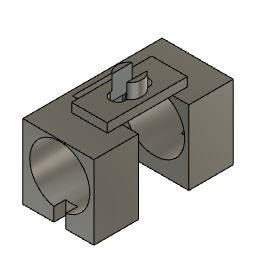
ENG_CRNK_mount-v2 v2-.25mm (Autodesk Fusion 360 design; units mm, degrees)
Autodesk Fusion 360 part; units mm, degrees
sketch "Sketch1" plane through (0, 0, 0) normal (0, 0, 1) x (1, 0, 0)
  line L0 (-39.3784, 42.4452) -> (-27.3784, 42.4452)
  line L1 (-27.3784, 42.4452) -> (-27.3784, 15.4452)
  line L2 (-27.3784, 15.4452) -> (-39.3784, 15.4452)
  line L3 (-39.3784, 15.4452) -> (-39.3784, 42.4452)
  dimension "d1" = 12
  dimension "d2" = 27
  constraint horizontal L0
  constraint vertical L1
  constraint horizontal L2
  constraint vertical L3
  measures "d1" distance of L0.start L0.end
  measures "d2" distance of L0.start L2.end
extrude "Extrude1" add sketch "Sketch1" along normal blind 3
sketch "Sketch2" plane through (0, 0, 3) normal (0, 0, 1) x (-1, 0, 0)
  line L0 (39.3784, -15.4452) -> (27.3784, -15.4452)
  line L1 (27.3784, -15.4452) -> (27.3784, -42.4452)
  line L2 (27.3784, -42.4452) -> (39.3784, -42.4452)
  line L3 (39.3784, -42.4452) -> (39.3784, -15.4452)
  circle A0 centre (33.3784, -28.9452) radius 4.25
  dimension "d5" = 8.5
  measures "d5" diameter of A0
extrude "Extrude2" add sketch "Sketch2" along normal blind 4.5 contours A0
sketch "Sketch3" plane through (0, 0, 0) normal (0, 0, -1) x (1, 0, 0)
  line L0 (-27.3784, -15.4452) -> (-39.3784, -15.4452)
  line L1 (-39.3784, -15.4452) -> (-39.3784, -42.4452)
  line L2 (-39.3784, -42.4452) -> (-27.3784, -42.4452)
  line L3 (-27.3784, -42.4452) -> (-27.3784, -15.4452)
  line L4 (-33.3784, -15.4452) -> (-30.8784, -15.4452) construction
  line L5 (-30.8784, -15.4452) -> (-35.8784, -15.4452)
  line L6 (-35.8784, -15.4452) -> (-35.8784, -42.4452)
  line L7 (-35.8784, -42.4452) -> (-30.8784, -42.4452)
  line L8 (-30.8784, -42.4452) -> (-30.8784, -15.4452)
  line L9 (-30.8784, -28.9452) -> (-30.8784, -24.9452) construction
  line L10 (-30.8784, -24.9452) -> (-35.8784, -24.9452)
  line L11 (-35.8784, -24.9452) -> (-35.8784, -32.9452)
  line L12 (-35.8784, -32.9452) -> (-30.8784, -32.9452)
  line L13 (-30.8784, -32.9452) -> (-30.8784, -24.9452)
  circle A0 centre (-33.3784, -32.9452) radius 2.5
  circle A1 centre (-33.3784, -24.9452) radius 2.5
  dimension "d8" = 2.5
  dimension "d9" = 5
  dimension "d10" = 4
  dimension "d11" = 8
  constraint midpoint L0 L4.start
  constraint perpendicular L3 L4
  constraint horizontal L5
  constraint vertical L6
  constraint horizontal L7
  constraint vertical L8
  constraint coincident L2 L6.end
  constraint midpoint L8 L9.start
  constraint coincident L8 L9.end
  constraint horizontal L10
  constraint vertical L11
  constraint horizontal L12
  constraint vertical L13
  constraint midpoint L12 A0.centre
  constraint coincident L12.end A0
  constraint midpoint L10 A1.centre
  constraint coincident L9.end A1
  measures "d8" distance of L4.start L4.end
  measures "d9" distance of L4.end L5.end
  measures "d10" distance of L9.start L9.end
  measures "d11" distance of L9.end L12.end
extrude "Extrude3" cut sketch "Sketch3" against normal blind 15 contours L10 A1 | L10 A1 | L6 L8 L11 L13 A0 A1 | L12 A0 | L12 A0
sketch "Sketch4" plane through (-35.8784, 0, 0) normal (1, 0, 0) x (0, 1, 0)
  line L0 (25.5083, 3) -> (24.9452, 3)
  line L1 (24.9452, 3) -> (24.9452, 0)
  line L2 (24.9452, 0) -> (32.9452, 0)
  line L3 (32.9452, 0) -> (32.9452, 3)
  line L4 (32.9452, 3) -> (32.3821, 3)
  line L5 (32.3821, 3) -> (32.3821, 7.5)
  line L6 (32.3821, 7.5) -> (25.5083, 7.5)
  line L7 (25.5083, 7.5) -> (25.5083, 3)
sketch "Sketch5" plane through (0, 0, 0) normal (0, 0, -1) x (1, 0, 0)
  line L0 (-35.8784, -32.9452) -> (-35.8784, -24.9452)
  arc A0 (-30.8784, -24.9452) -> (-35.8784, -24.9452) centre (-33.3784, -24.9452) ccw
  line L1 (-30.8784, -24.9452) -> (-30.8784, -32.9452)
  arc A1 (-35.8784, -32.9452) -> (-30.8784, -32.9452) centre (-33.3784, -32.9452) ccw
  line L2 (-27.3784, -15.4452) -> (-39.3784, -15.4452)
  line L3 (-39.3784, -15.4452) -> (-39.3784, -42.4452)
  line L4 (-39.3784, -42.4452) -> (-27.3784, -42.4452)
  line L5 (-27.3784, -42.4452) -> (-27.3784, -15.4452)
  line L6 (-39.3784, -42.4452) -> (-27.3784, -42.4452)
  line L7 (-27.3784, -42.4452) -> (-27.3784, -38.4452)
  line L8 (-27.3784, -38.4452) -> (-39.3784, -38.4452)
  line L9 (-39.3784, -38.4452) -> (-39.3784, -42.4452)
  line L10 (-39.3784, -15.4452) -> (-27.3784, -15.4452)
  line L11 (-27.3784, -15.4452) -> (-27.3784, -19.4452)
  line L12 (-27.3784, -19.4452) -> (-39.3784, -19.4452)
  line L13 (-39.3784, -19.4452) -> (-39.3784, -15.4452)
  dimension "d14" = 4
  dimension "d15" = 4
  constraint horizontal L6
  constraint vertical L7
  constraint horizontal L8
  constraint vertical L9
  constraint coincident L3.end L4.start
  constraint horizontal L10
  constraint vertical L11
  constraint horizontal L12
  constraint vertical L13
  constraint coincident L5 L11.end
  constraint coincident L2.end L3.start
  measures "d14" distance of L3.end L8.end
  measures "d15" distance of L2.end L12.end
extrude "Extrude4" add sketch "Sketch5" along normal blind 25 contours L2 L3 L5 L10 L11 L12 L13 | L3 L4 L5 L6 L7 L8 L9
sketch "Sketch6" plane through (-27.3784, 0, 0) normal (1, 0, 0) x (0, 1, 0)
  line L0 (42.4452, -25) -> (42.4452, 3)
  line L1 (42.4452, 3) -> (15.4452, 3)
  line L2 (15.4452, 3) -> (15.4452, -25)
  line L3 (15.4452, -25) -> (19.4452, -25)
  line L4 (19.4452, -25) -> (19.4452, 0)
  line L5 (19.4452, 0) -> (38.4452, 0)
  line L6 (38.4452, 0) -> (38.4452, -25)
  line L7 (38.4452, -25) -> (42.4452, -25)
  line L8 (19.4452, 0) -> (15.4452, 0)
  line L9 (38.4452, 0) -> (42.4452, 0)
  constraint coincident L4.end L5.start
  constraint coincident L2 L8.end
  constraint perpendicular L2 L8
  constraint coincident L5.end L6.start
  constraint coincident L0 L9.end
  constraint perpendicular L0 L9
extrude "Extrude5" add sketch "Sketch6" along normal blind 4 contours L0 L6 L7 L9 | L2 L3 L4 L8
sketch "Sketch7" plane through (-39.3784, 0, 0) normal (-1, 0, 0) x (0, -1, 0)
  line L0 (-15.4452, -25) -> (-15.4452, 3)
  line L1 (-15.4452, 3) -> (-42.4452, 3)
  line L2 (-42.4452, 3) -> (-42.4452, -25)
  line L3 (-42.4452, -25) -> (-38.4452, -25)
  line L4 (-38.4452, -25) -> (-38.4452, 0)
  line L5 (-38.4452, 0) -> (-19.4452, 0)
  line L6 (-19.4452, 0) -> (-19.4452, -25)
  line L7 (-19.4452, -25) -> (-15.4452, -25)
  line L8 (-42.4452, 0) -> (-15.4452, 0)
  constraint coincident L2 L8.start
  constraint coincident L0 L8.end
  constraint perpendicular L0 L8
extrude "Extrude6" add sketch "Sketch7" along normal blind 4 contours L0 L6 L7 L8 | L2 L3 L4 L8
sketch "Sketch8" plane through (0, 15.4452, 0) normal (0, -1, 0) x (1, 0, 0)
  line L0 (-27.3784, 0) -> (-27.3784, 3)
  line L1 (-27.3784, 3) -> (-39.3784, 3)
  line L2 (-39.3784, 3) -> (-39.3784, 0)
  line L3 (-39.3784, 0) -> (-43.3784, 0)
  line L4 (-43.3784, 0) -> (-43.3784, -25)
  line L5 (-43.3784, -25) -> (-23.3784, -25)
  line L6 (-23.3784, -25) -> (-23.3784, 0)
  line L7 (-23.3784, 0) -> (-27.3784, 0)
  line L8 (-39.3784, 0) -> (-27.3784, 0)
  constraint coincident L2.end L3.start
  constraint coincident L0.start L7.end
extrude "Extrude7" add sketch "Sketch8" along normal blind 11 contours L3 L4 L5 L6 L7 L8
sketch "Sketch9" plane through (0, 42.4452, 0) normal (0, 1, 0) x (-1, 0, 0)
  line L0 (39.3784, 0) -> (39.3784, 3)
  line L1 (39.3784, 3) -> (27.3784, 3)
  line L2 (27.3784, 3) -> (27.3784, 0)
  line L3 (27.3784, 0) -> (23.3784, 0)
  line L4 (23.3784, 0) -> (23.3784, -25)
  line L5 (23.3784, -25) -> (43.3784, -25)
  line L6 (43.3784, -25) -> (43.3784, 0)
  line L7 (43.3784, 0) -> (39.3784, 0)
  line L8 (27.3784, 0) -> (39.3784, 0)
  constraint coincident L2.end L3.start
  constraint coincident L0.start L7.end
extrude "Extrude8" add sketch "Sketch9" along normal blind 11 contours L3 L4 L5 L6 L7 L8
sketch "Sketch10" plane through (0, 53.4452, 0) normal (0, 1, 0) x (-1, 0, 0)
  line L0 (23.3784, 0) -> (23.3784, -25)
  line L1 (23.3784, -25) -> (43.3784, -25)
  line L2 (43.3784, -25) -> (43.3784, 0)
  line L3 (43.3784, 0) -> (23.3784, 0)
  line L4 (33.3784, 0) -> (33.3784, -10.5) construction
  circle A0 centre (33.3784, -10.5) radius 10
  dimension "d26" = 10.5
  dimension "d27" = 20
  constraint midpoint L3 L4.start
  constraint perpendicular L3 L4
  constraint coincident L4.end A0.centre
  measures "d26" distance of L4.start L4.end
  measures "d27" diameter of A0
extrude "Extrude9" cut sketch "Sketch10" against normal blind 62 contours A0
extrude "Extrude10" add 4 faces at (-23.3784, 48.4452, -3.5) (-23.3784, 9.4452, -7) (-23.3784, 14.4452, -20.1667) (-23.3784, 48.4452, -20.1667) along direction (1, 0, 0) blind 0.5
extrude "Extrude11" add 4 faces at (-43.3784, 43.4452, -3.5) (-43.3784, 48.4452, -20.1667) (-43.3784, 14.4452, -15.3333) (-43.3784, 14.4452, -3.5) along direction (-1, 0, 0) blind 0.5
extrude "Extrude12" add 1 faces at (-33.1293, 38.4452, -23.4907) along direction (0, -1, 0) blind 1
extrude "Extrude13" add 1 faces at (-33.1293, 19.4452, -23.4907) along direction (0, 1, 0) blind 1
extrude "Extrude14" add 1 faces at (-43.8784, 42.7785, -8.3333) along direction (-1, 0, 0) blind 2
extrude "Extrude15" add 1 faces at (-43.8784, 15.1119, -8.3333) along direction (-1, 0, 0) blind 2
extrude "Extrude16" add 1 faces at (-22.8784, 42.7785, -16.6667) along direction (1, 0, 0) blind 2
extrude "Extrude17" add 1 faces at (-22.8784, 15.1119, -8.3333) along direction (1, 0, 0) blind 2
extrude "Extrude18" cut 1 faces at (-33.1293, 4.4452, -23.4907) along direction (0, 1, 0) blind 1
extrude "Extrude19" cut 1 faces at (-33.1293, 53.4452, -23.4907) along direction (0, -1, 0) blind 1
extrude "Extrude20" add 2 faces at (-30.1717, 28.772, 7.5) (-36.576, 27.9712, 7.5) along direction (0, 0, 1) blind 0.5
sketch "Sketch11" plane through (0, 52.4452, 0) normal (0, 1, 0) x (-1, 0, 0)
  line L0 (45.8784, 0) -> (20.8784, 0)
  line L1 (20.8784, 0) -> (20.8784, -25)
  line L2 (20.8784, -25) -> (45.8784, -25)
  line L3 (45.8784, -25) -> (45.8784, 0)
  circle A0 centre (33.3784, -10.5) radius 10
  line L4 (45.8784, 0) -> (44.1284, 0)
  line L5 (44.1284, 0) -> (44.1284, -25)
  line L6 (44.1284, -25) -> (45.8784, -25)
  line L7 (45.8784, -25) -> (45.8784, 0)
  dimension "d52" = 1.75
  constraint horizontal L4
  constraint vertical L5
  constraint horizontal L6
  constraint vertical L7
  constraint coincident L2 L5.end
  constraint coincident L0.start L3.end
  measures "d52" distance of L0.start L4.end
extrude "Extrude21" add sketch "Sketch11" against normal blind 47 contours L0 L2 L3 L4 L5 L6 L7
extrude "Extrude22" cut 2 faces at (-20.8784, 47.4452, -16.6667) (-20.8784, 10.4452, -8.3333) along direction (-1, 0, 0) blind 1
sketch "Sketch12" plane through (0, 52.4452, 0) normal (0, 1, 0) x (-1, 0, 0)
  line L0 (21.8784, 0) -> (21.8784, -25)
  line L1 (21.8784, -25) -> (45.8784, -25)
  line L2 (45.8784, -25) -> (45.8784, 0)
  line L3 (45.8784, 0) -> (21.8784, 0)
  circle A0 centre (33.3784, -10.5) radius 10
  circle A1 centre (33.3784, -10.5) radius 10.125
  dimension "d67" = 20.25
  constraint concentric A0 A1
  measures "d67" diameter of A1
extrude "Extrude25" cut sketch "Sketch12" against normal blind 68 contours A1
sketch "Sketch13" plane through (0, 0, -25) normal (0, 0, -1) x (1, 0, 0)
  line L0 (-21.8784, -52.4452) -> (-21.8784, -37.4452)
  line L1 (-21.8784, -37.4452) -> (-44.1284, -37.4452)
  line L2 (-44.1284, -37.4452) -> (-44.1284, -20.4452)
  line L3 (-44.1284, -20.4452) -> (-21.8784, -20.4452)
  line L4 (-21.8784, -20.4452) -> (-21.8784, -5.4452)
  line L5 (-21.8784, -5.4452) -> (-45.8784, -5.4452)
  line L6 (-45.8784, -5.4452) -> (-45.8784, -52.4452)
  line L7 (-45.8784, -52.4452) -> (-21.8784, -52.4452)
  line L8 (-45.8784, -52.4452) -> (-33.3784, -52.4452) construction
  line L9 (-33.3784, -52.4452) -> (-35.3784, -52.4452) construction
  line L10 (-35.3784, -52.4452) -> (-31.3784, -52.4452)
  line L11 (-31.3784, -52.4452) -> (-31.3784, -48.4452)
  line L12 (-31.3784, -48.4452) -> (-35.3784, -48.4452)
  line L13 (-35.3784, -48.4452) -> (-35.3784, -52.4452)
  dimension "d57" = 12.5
  dimension "d58" = 2
  dimension "d59" = 4
  dimension "d60" = 4
  constraint coincident L6.end L7.start
  constraint coincident L7 L8.end
  constraint parallel L8 L9
  constraint horizontal L10
  constraint vertical L11
  constraint horizontal L12
  constraint vertical L13
  measures "d57" distance of L6.end L8.end
  measures "d58" distance of L8.end L9.end
  measures "d59" distance of L9.end L10.end
  measures "d60" distance of L9.end L12.end
extrude "Extrude23" cut sketch "Sketch13" against normal blind 10 contours L7 L10 L11 L12 L13
sketch "Sketch14" plane through (0, 0, -25) normal (0, 0, -1) x (1, 0, 0)
  line L0 (-35.3784, -52.4452) -> (-35.3784, -48.4452)
  line L1 (-35.3784, -48.4452) -> (-31.3784, -48.4452)
  line L2 (-31.3784, -48.4452) -> (-31.3784, -52.4452)
  line L3 (-31.3784, -52.4452) -> (-21.8784, -52.4452)
  line L4 (-21.8784, -52.4452) -> (-21.8784, -37.4452)
  line L5 (-21.8784, -37.4452) -> (-44.1284, -37.4452)
  line L6 (-44.1284, -37.4452) -> (-44.1284, -20.4452)
  line L7 (-44.1284, -20.4452) -> (-21.8784, -20.4452)
  line L8 (-21.8784, -20.4452) -> (-21.8784, -5.4452)
  line L9 (-21.8784, -5.4452) -> (-45.8784, -5.4452)
  line L10 (-45.8784, -5.4452) -> (-45.8784, -52.4452)
  line L11 (-45.8784, -52.4452) -> (-35.3784, -52.4452)
  line L12 (-35.3784, -48.4452) -> (-35.3784, -5.4452) construction
  line L13 (-35.3784, -5.4452) -> (-31.3784, -5.4452)
  line L14 (-31.3784, -5.4452) -> (-31.3784, -9.4452)
  line L15 (-31.3784, -9.4452) -> (-35.3784, -9.4452)
  line L16 (-35.3784, -9.4452) -> (-35.3784, -5.4452)
  dimension "d63" = 4
  dimension "d64" = 4
  constraint coincident L0.end L1.start
  constraint coincident L9 L12.end
  constraint perpendicular L9 L12
  constraint horizontal L13
  constraint vertical L14
  constraint horizontal L15
  constraint vertical L16
  measures "d63" distance of L12.end L13.end
  measures "d64" distance of L12.end L15.end
extrude "Extrude24" cut sketch "Sketch14" against normal blind 7 contours L9 L13 L14 L15 L16
